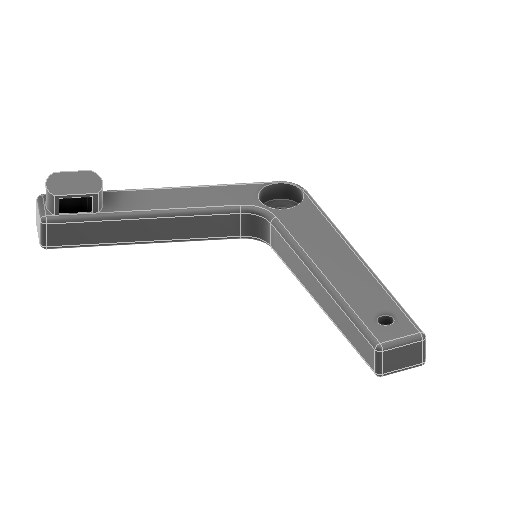
# Autodesk Inventor part: bogie
Saved by Autodesk Inventor 2025 (Build 290162010, 162A)
## iProperties
Created: 2024-08-06
Part Number: bogie
Material: Generic
Document SubType Name: Modeling
Designer: Pauline Simonnet
Density: 1 g/cm^3
Appearance: Smooth - Black
Author: Pauline Simonnet
Autodesk Inventor part; units mm, degrees
ref_plane "YZ Plane" through (0, 0, 0) normal (1, 0, 0) x (0, 1, 0)
ref_plane "XZ Plane" through (0, 0, 0) normal (0, 1, 0) x (-1, 0, 0)
ref_plane "XY Plane" through (0, 0, 0) normal (0, 0, 1) x (1, 0, 0)
sketch "Sketch1" plane through (0, 0, 0) normal (0, 1, 0) x (-1, 0, 0)
  line L0 (-449.3983, -167.7502) -> (-378.3636, -81.8866)
  line L1 (-378.3636, -81.8866) -> (-449.3983, -167.7502)
  line L2 (-449.3983, -167.7502) -> (-576.7175, -122.4118)
  line L3 (-576.7175, -122.4118) -> (-586.1106, -148.7893)
  line L4 (-586.1106, -148.7893) -> (-444.3316, -199.2768)
  line L5 (-378.3636, -81.8866) -> (-359.8715, -97.185)
  line L6 (-359.8715, -97.185) -> (-444.3316, -199.2768)
  line L7 (-444.3316, -199.2768) -> (-443.437, -196.7644) construction
  line L8 (-444.3316, -199.2768) -> (-472.9863, -175.5709) construction
  circle A0 centre (-449.1927, -181.6278) radius 4.4
  circle A1 centre (-562.573, -142.3098) radius 4.3
  line L9 (-369.4222, -102.8465) -> (-379.0472, -114.4809)
  line L10 (-381.7502, -92.6476) -> (-391.3753, -104.2819)
  line L11 (-374.2347, -108.6637) -> (-386.5628, -98.4648) construction
  line L12 (-369.1175, -89.5358) -> (-380.3987, -103.5642) construction
  arc A2 (-369.4222, -102.8465) -> (-381.7502, -92.6476) centre (-380.3987, -103.5642) ccw
  arc A3 (-391.3753, -104.2819) -> (-379.0472, -114.4809) centre (-380.3987, -103.5642) ccw
  point P0 (0, 0)
  dimension "d17" = 110
  dimension "d18" = 28
  dimension "d19" = 24
  dimension "d20" = 90
  dimension "d21" = 90
  dimension "d23" = 8.6
  dimension "d24" = 8.8
  dimension "d25" = 20
  dimension "d26" = 14
  dimension "d29" = 10.5
  dimension "d30" = 10.5
  dimension "d31" = 140
  dimension "d32" = 122
  dimension "d43" = 16
  dimension "d44" = 4.25
  dimension "d46" = 11
  dimension "d47" = 18
  dimension "d65" = 182.1743
  constraints: 26 end point, 4 centre point, 4 midpoint, 4 point on circle, 1 coincident, 1 collinear, 1 perpendicular
  measures "d17" angle of L2 L0
  measures "d18" distance between parallel lines of L4 L2
  measures "d19" distance between parallel lines of L0 L6
  measures "d20" angle of L8 L6
  measures "d21" angle of L4 L7
  measures "d23" diameter of A1
  measures "d24" diameter of A0
  measures "d25" distance from line of L3 A1.centre
  measures "d26" distance from line of A1.centre L2
  measures "d29" distance from line of A0.centre L7
  measures "d30" distance from line of L8 A0.centre
  measures "d31" distance from line of L3 A0.centre
  measures "d32" distance from line of A0.centre L5
  measures "d43" distance between parallel lines of L10 L9
  measures "d44" distance between parallel lines of L0 L10
  measures "d46" radius of A3
  measures "d47" distance between parallel lines of L11 L5
  measures "d65" horizontal distance of L12.end A1.centre
extrude "Extrusion1" add sketch "Sketch1" along normal blind 20
fillet "Fillet1" radius 15 1 edges at (449.3983, 10, -167.7502)
fillet "Fillet2" radius 15 1 edges at (444.3316, 10, -199.2768)
fillet "Fillet3" radius 3 2 edges at (518.0051, 20, -143.3193) (410.5334, 20, -120.7721)
fillet "Fillet4" radius 3 3 edges at (445.211, 20, -196.0841) (520.1683, 20, -172.2713) (398.754, 20, -144.1846)
fillet "Fillet5" radius 3 3 edges at (445.211, 0, -196.0841) (520.1683, 0, -172.2713) (398.754, 0, -144.1846)
fillet "Fillet6" radius 3 2 edges at (518.0051, 0, -143.3193) (410.5334, 0, -120.7721)
fillet "Fillet7" radius 3 8 edges at (585.8158, 19.1213, -147.9615) (581.414, 20, -135.6005) (577.0123, 19.1213, -123.2396) (576.7175, 10, -122.4118) (577.0123, 0.8787, -123.2396) (581.414, 0, -135.6005) (585.8158, 0.8787, -147.9615) (586.1106, 10, -148.7893)
fillet "Fillet8" radius 3 8 edges at (377.6865, 0.8787, -82.4467) (378.3636, 10, -81.8866) (377.6865, 19.1213, -82.4467) (369.1175, 20, -89.5358) (360.5485, 19.1213, -96.6249) (359.8715, 10, -97.185) (360.5485, 0.8787, -96.6249) (369.1175, 0, -89.5358)
sketch "Sketch2" plane through (0, 20, 0) normal (0, 1, 0) x (1, 0, 0)
  arc A0 (391.3753, 104.2819) -> (379.0472, 114.4809) centre (380.3987, 103.5642) ccw projected
  arc A1 (369.4222, 102.8465) -> (381.7502, 92.6476) centre (380.3987, 103.5642) ccw projected
  line L0 (377.9644, 86.1104) -> (440.3917, 161.5699) projected
  line L1 (380.5955, 89.2908) -> (394.732, 106.3784)
  line L2 (367.9947, 102.6898) -> (378.9337, 115.9125)
  line L3 (369.4222, 102.8465) -> (379.0472, 114.4809) projected
  line L4 (366.124, 103.5662) -> (378.0493, 117.981)
  arc A2 (366.124, 103.5662) -> (380.5955, 89.2908) centre (380.3987, 103.5642) ccw
  arc A3 (394.732, 106.3784) -> (378.0493, 117.981) centre (380.3987, 103.5642) ccw
  arc A4 (367.9947, 102.6898) -> (382.2286, 91.2648) centre (380.3987, 103.5642) ccw
  arc A5 (392.8232, 104.0711) -> (378.9337, 115.9125) centre (380.3987, 103.5642) ccw
  point P0 (0, 0)
  point P1 (392.8232, 104.0711)
  point P2 (382.2286, 91.2648)
  dimension "d48" = 0
  dimension "d49" = 0
  dimension "d53" = 1
  dimension "d54" = 2
  constraints: 8 point on circle, 6 end point, 4 centre point, 4 point on line, 2 parallel, 1 coincident
  measures "d48" distance of A0.centre A4.centre
  measures "d49" distance of A4.centre A0.centre
  measures "d53" distance between parallel lines of L3 L2
  measures "d54" distance between parallel lines of L2 L4
extrude "Extrusion2" add sketch "Sketch2" along normal blind 10 contours A2 L4 A3 L0 A5 L2 A4
sketch "Sketch3" plane through (0, 30, 0) normal (0, 1, 0) x (1, 0, 0)
  line L0 (382.2286, 91.2648) -> (380.5955, 89.2908) projected
  arc A0 (394.732, 106.3784) -> (381.1124, 118.1537) centre (380.3987, 103.5642) ccw projected
  line L1 (380.5955, 89.2908) -> (394.732, 106.3784)
  line L2 (378.0493, 117.981) -> (366.124, 103.5662) projected
  line L3 (366.124, 103.5662) -> (378.0493, 117.981)
  arc A1 (366.124, 103.5662) -> (380.5955, 89.2908) centre (380.3987, 103.5642) ccw
  arc A2 (394.732, 106.3784) -> (378.0493, 117.981) centre (380.3987, 103.5642) ccw
  point P0 (0, 0)
  constraints: 4 end point, 4 point on circle, 2 centre point, 1 coincident, 1 collinear
extrude "Extrusion3" add sketch "Sketch3" along normal blind 2
fillet "Fillet9" radius 2 1 edges at (372.0866, 20, -110.7736)
sketch "Sketch4" plane through (0, 20, 0) normal (0, 1, 0) x (1, 0, 0)
  circle A0 centre (449.1927, 181.6278) radius 11.425
  circle A1 centre (449.1927, 181.6278) radius 4.4 projected
  point P0 (0, 0)
  dimension "d60" = 0
  dimension "d61" = 0
  dimension "d62" = 22.85
  constraints: 1 centre point
  measures "d60" distance of A1.centre A0.centre
  measures "d61" distance of A1.centre A0.centre
  measures "d62" diameter of A0
extrude "Extrusion4" cut sketch "Sketch4" against normal blind 10
sketch "Schizzo5" plane through (239.9307, 0, -245.6335) normal (0, -1, 0) x (1, 0, 0)
  circle A0 centre (447.9395, 177.9208) radius 11.425
  circle A1 centre (447.9395, 177.9208) radius 4.4
  point P0 (0, 0)
  dimension "d68" = 0
  dimension "d67" = 0
  dimension "d66" = 22.85
  constraints: 2 centre point
  measures "d68" distance of A1.centre A0.centre
  measures "d67" distance of A1.centre A0.centre
  measures "d66" diameter of A0
extrude "Estrusione5" cut sketch "Schizzo5" against normal blind 10
sketch "Schizzo6" plane through (0, 0, 0) normal (0, -1, 0) x (1, 0, 0)
  circle A0 centre (562.573, -142.3098) radius 4.3 projected
  circle A1 centre (562.573, -142.3098) radius 11.425
  point P0 (0, 0)
  dimension "d72" = 22.85
  constraints: 1 centre point, 1 coincident
  measures "d72" diameter of A1
extrude "Estrusione6" cut sketch "Schizzo6" against normal blind 10 contours A0 | A1
body "Solid1"
